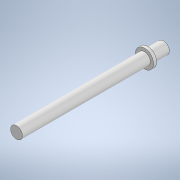
# Autodesk Inventor part: reverser-base
Saved by Autodesk Inventor 2021 (Build 250183000, 183)
## iProperties
Created: 2021-07-09
Part Number: reverser-base
Material: Generic
Document SubType Name: Modeling
Designer: teh18
Density: 1 g/cm^3
Appearance: Default
Author: teh18
Autodesk Inventor part; units mm, degrees
ref_plane "YZ Plane" through (0, 0, 0) normal (1, 0, 0) x (0, 1, 0)
ref_plane "XZ Plane" through (0, 0, 0) normal (0, 1, 0) x (-1, 0, 0)
ref_plane "XY Plane" through (0, 0, 0) normal (0, 0, 1) x (1, 0, 0)
sketch "Sketch1" plane through (0, 0, 0) normal (0, 0, 1) x (1, 0, 0)
  line L0 (3, -1) -> (-3, -1) projected
  line L1 (-3, -1) -> (-3, 1) projected
  line L2 (-3, 1) -> (3, 1) projected
  line L3 (3, 1) -> (3, -1) projected
  circle A0 centre (0, 0) radius 3.75 projected
  line L4 (-3.1, 1.1) -> (-3.1, -1.1)
  line L5 (-3.1, -1.1) -> (3.1, -1.1)
  line L6 (3.1, -1.1) -> (3.1, 1.1)
  line L7 (3.1, 1.1) -> (-3.1, 1.1)
  circle A1 centre (0, 0) radius 5.75
  dimension "d0" = 0.1
  dimension "d5" = 2
  constraints: 8 end point, 1 centre point, 3 other
  measures "d0" distance between parallel lines of L1 L4
  measures "d5" radial gap between concentric circles of A0 A1
extrude "Extrusion1" add sketch "Sketch1" along normal blind 10 contours A0 | A1
sketch "Sketch2" plane through (0, 0, 10) normal (0, 0, 1) x (1, 0, 0)
  line L0 (-3.1, 1.1) -> (3.1, 1.1) projected
  line L1 (3.1, 1.1) -> (3.1, -1.1) projected
  line L2 (3.1, -1.1) -> (-3.1, -1.1) projected
  line L3 (-3.1, -1.1) -> (-3.1, 1.1) projected
  circle A0 centre (0, 0) radius 3.75
  constraints: 1 centre point
ref_plane "Work Plane1" through (-14, -11, 93) normal (0, 0, -1) x (0, 1, 0)
extrude "Extrusion2" add sketch "Sketch2" along normal up to surface (83 mm away) contours L0 L1 L2 L3 | A0
body "Solid1"
